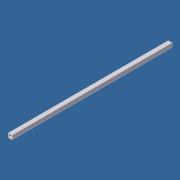
# Autodesk Inventor part: GE-12016-05
Saved by Autodesk Inventor 2012 (Build 160160000, 160)
## iProperties
Created: 2011-09-23
Part Number: GE-12016-05
Document SubType Name: Modeling
Designer: dfoster
Density: 2.71 g/cm^3
Material: Aluminum-6061
Mass: 2561.84 g
Surface Area: 5965.31 cm^2
Volume: 945.329 cm^3
Description: Middle Horizontal
Title: Middle Horizontal
Author: dfoster
Autodesk Inventor part; units mm, degrees
ref_plane "YZ Plane" through (0, 0, 0) normal (1, 0, 0) x (0, 1, 0)
ref_plane "XZ Plane" through (0, 0, 0) normal (0, 1, 0) x (-1, 0, 0)
ref_plane "XY Plane" through (0, 0, 0) normal (0, 0, 1) x (1, 0, 0)
sketch "Sketch1" plane through (0, 0, 0) normal (0, 0, 1) x (1, 0, 0)
  line L0 (0, 0) -> (44.45, 0)
  line L1 (44.45, 0) -> (44.45, 44.45)
  line L2 (44.45, 44.45) -> (0, 44.45)
  line L3 (0, 44.45) -> (0, 0)
  line L4 (3.175, 41.275) -> (41.275, 41.275)
  line L5 (41.275, 41.275) -> (41.275, 3.175)
  line L6 (41.275, 3.175) -> (3.175, 3.175)
  line L7 (3.175, 3.175) -> (3.175, 41.275)
  dimension "d0" = 3.175
  dimension "d1" = 44.45
  constraints: 16 end point, 4 parallel, 3 perpendicular, 1 horizontal, 3 other
  measures "d0" distance between parallel lines of L4 L2
  measures "d1" distance of L1.end L2.end
extrude "Extrusion1" add sketch "Sketch1" along normal blind 1803.4
body "Solid1"
